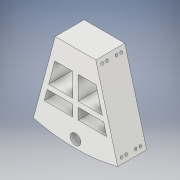
# Autodesk Inventor part: CA001
Saved by Autodesk Inventor 2017 SP1 (Build 210196100, 196)
## iProperties
Created: 2017-06-04
Part Number: CA001
Material: ABS Plastic
Document SubType Name: Modeling
Designer: Zach
Density: 1.06 g/cm^3
Appearance: CR White
Author: Zach
Autodesk Inventor part; units mm, degrees
ref_plane "YZ Plane" through (0, 0, 0) normal (1, 0, 0) x (0, 1, 0)
ref_plane "XZ Plane" through (0, 0, 0) normal (0, 1, 0) x (-1, 0, 0)
ref_plane "XY Plane" through (0, 0, 0) normal (0, 0, 1) x (1, 0, 0)
sketch "Sketch1" plane through (0, 0, 0) normal (0, 0, 1) x (1, 0, 0)
  line L0 (0, 0) -> (160, 0)
  line L1 (160, 0) -> (118.589, 154.5481)
  line L2 (41.411, 154.5481) -> (0, 0)
  line L3 (41.411, 154.5481) -> (118.589, 154.5481)
  dimension "d0" = 160
  dimension "d1" = 160
  dimension "d2" = 75
  dimension "d8" = 75
  constraints: 8 end point, 2 horizontal
  measures "d0" distance of L0.start L0.end
  measures "d1" distance of L1.end L0.end
  measures "d2" angle of L1 L0
  measures "d8" angle of L0 L2
extrude "Extrusion1" add sketch "Sketch1" along normal blind 55
sketch "Sketch6" plane through (0, 0, 55) normal (0, 0, 1) x (1, 0, 0)
  line L0 (0, 0) -> (160, 0) construction
  line L1 (160, 0) -> (118.589, 154.5481) construction
  line L2 (118.589, 154.5481) -> (41.411, 154.5481) construction
  line L3 (41.411, 154.5481) -> (0, 0) construction
  line L4 (110.9157, 144.5481) -> (146.9677, 10) construction
  line L5 (146.9677, 10) -> (13.0323, 10) construction
  line L6 (13.0323, 10) -> (49.0843, 144.5481) construction
  line L7 (49.0843, 144.5481) -> (110.9157, 144.5481) construction
  line L8 (85, 144.5481) -> (75, 144.5481) construction
  line L9 (75, 144.5481) -> (75, 10) construction
  line L10 (75, 10) -> (85, 10) construction
  line L11 (85, 10) -> (85, 144.5481) construction
  line L12 (133.5703, 60) -> (26.4297, 60) construction
  line L13 (26.4297, 60) -> (26.4297, 70) construction
  line L14 (26.4297, 70) -> (133.5703, 70) construction
  line L15 (133.5703, 70) -> (133.5703, 60) construction
  line L16 (133.5703, 60) -> (146.9677, 10)
  line L17 (85, 10) -> (146.9677, 10)
  line L18 (0, 0) -> (160, 0) construction
  line L19 (133.5703, 60) -> (85, 60)
  line L20 (85, 60) -> (85, 10)
  line L21 (75, 10) -> (75, 60)
  line L22 (26.4297, 60) -> (75, 60)
  line L23 (26.4297, 60) -> (13.0323, 10)
  line L24 (13.0323, 10) -> (75, 10)
  line L25 (75, 70) -> (75, 144.5481)
  line L26 (75, 144.5481) -> (49.0843, 144.5481)
  line L27 (75, 70) -> (29.1092, 70)
  line L28 (29.1092, 70) -> (49.0843, 144.5481)
  line L29 (85, 144.5481) -> (110.9157, 144.5481)
  line L30 (110.9157, 144.5481) -> (130.8908, 70)
  line L31 (130.8908, 70) -> (85, 70)
  line L32 (85, 70) -> (85, 144.5481)
  point P0 (80, 10)
  dimension "d22" = 10
  dimension "d23" = 10
  dimension "d24" = 10
  dimension "d25" = 50
  constraints: 56 end point, 16 point on line, 6 collinear, 6 parallel, 3 perpendicular, 2 horizontal, 2 midpoint, 3 other
  measures "d22" distance between parallel lines of L1 L4
  measures "d23" distance between parallel lines of L9 L11
  measures "d24" distance of L12.end L13.end
  measures "d25" distance between parallel lines of L5 L12
extrude "Extrusion5" cut sketch "Sketch6" against normal through all
sketch "Sketch7" plane through (0, 0, 0) normal (0, 0, -1) x (-1, 0, 0)
  circle A0 centre (-80, 304.672) radius 315 construction
  line L0 (0, 0) -> (-160, 0) projected
  arc A1 (-160, 0) -> (0, 0) centre (-80, 304.672) ccw
  dimension "d28" = 630
  constraints: 4 point on circle, 2 centre point, 1 concentric
  measures "d28" diameter of A0
extrude "Extrusion6" add sketch "Sketch7" against normal blind 55
sketch "Sketch8" plane through (0, 0, 0) normal (0, 0, -1) x (-1, 0, 0)
  circle A0 centre (-80, 4.836) radius 10
  line L0 (-15.7117, 20) -> (-144.2883, 20) construction
  line L1 (-13.0323, 10) -> (-15.7117, 20)
  line L2 (-15.7117, 20) -> (-75, 20)
  line L3 (-75, 10) -> (-75, 60) projected
  line L4 (-75, 20) -> (-75, 10)
  line L5 (-75, 10) -> (-13.0323, 10) projected
  line L6 (-75, 10) -> (-13.0323, 10)
  line L7 (-26.4297, 60) -> (-13.0323, 10) projected
  line L8 (-85, 10) -> (-146.9677, 10) projected
  line L9 (-146.9677, 10) -> (-144.2883, 20)
  line L10 (-133.5703, 60) -> (-146.9677, 10) projected
  line L11 (-144.2883, 20) -> (-85, 20)
  line L12 (-85, 60) -> (-85, 10) projected
  line L13 (-85, 20) -> (-85, 10)
  line L14 (-85, 10) -> (-146.9677, 10)
  line L15 (-118.589, 154.5481) -> (-41.411, 154.5481) projected
  arc A1 (-160, 0) -> (0, 0) centre (-80, 304.672) ccw projected
  line L16 (0, -10.328) -> (-160, -10.328) construction
  arc A2 (-160, 0) -> (0, 0) centre (-80, 304.672) ccw projected
  line L17 (-0.263, 4.836) -> (-159.737, 4.836) construction
  point P0 (-80, 154.5481)
  dimension "d31" = 20
  dimension "d32" = 20
  constraints: 22 end point, 6 point on line, 4 collinear, 3 horizontal, 2 midpoint, 1 centre point, 1 coincident, 1 perpendicular, 1 tangent, 1 vertical alignment, 1 other
  measures "d31" diameter of A0
  measures "d32" distance from line of A1.end L0
extrude "Extrusion8" add sketch "Sketch8" against normal blind 55 contours L5 L3 A0 | A0 L3 L2 L1 L5 | L8 L9 L11 L12 A0 | A0 L12 L8
extrude "Extrusion7" cut sketch "Sketch8" against normal through all contours A0 L8 L12 L3 L5 | L5 L3 A0 | A0 L12 L8
sketch "Sketch14" plane through (15.7117, 20, 0) normal (0, 1, 0) x (1, 0, 0)
  line L0 (0, 0) -> (59.2883, 0) construction
  line L1 (0, -55) -> (0, 0) construction
  line L2 (59.2883, -55) -> (0, -55) construction
  line L3 (59.2883, 0) -> (59.2883, -55) construction
  line L4 (69.2883, 0) -> (128.5765, 0) construction
  line L5 (69.2883, -55) -> (69.2883, 0) construction
  line L6 (128.5765, -55) -> (69.2883, -55) construction
  line L7 (128.5765, 0) -> (128.5765, -55) construction
  circle A0 centre (118.9324, -7.5) radius 2.5
  circle A1 centre (78.9324, -7.5) radius 2.5
  circle A2 centre (78.9324, -47.5) radius 2.5
  circle A3 centre (118.9324, -47.5) radius 2.5
  line L8 (118.9324, -7.5) -> (78.9324, -7.5) construction
  line L9 (78.9324, -7.5) -> (78.9324, -47.5) construction
  line L10 (78.9324, -47.5) -> (118.9324, -47.5) construction
  line L11 (118.9324, -47.5) -> (118.9324, -7.5) construction
  line L12 (49.6441, -7.5) -> (9.6441, -7.5) construction
  line L13 (9.6441, -7.5) -> (9.6441, -47.5) construction
  line L14 (9.6441, -47.5) -> (49.6441, -47.5) construction
  line L15 (49.6441, -47.5) -> (49.6441, -7.5) construction
  circle A4 centre (49.6441, -7.5) radius 2.5
  circle A5 centre (9.6441, -7.5) radius 2.5
  circle A6 centre (9.6441, -47.5) radius 2.5
  circle A7 centre (49.6441, -47.5) radius 2.5
  point P0 (-15.7117, 0)
  point P1 (78.9324, -27.5)
  point P2 (98.9324, -7.5)
  point P3 (29.6441, -7.5)
  point P4 (49.6441, -27.5)
  dimension "d77" = 5
  dimension "d78" = 5
  dimension "d79" = 5
  dimension "d80" = 5
  dimension "d81" = 40
  dimension "d83" = 40
  dimension "d84" = 40
  dimension "d85" = 40
  dimension "d86" = 5
  dimension "d87" = 5
  dimension "d88" = 5
  dimension "d89" = 5
  constraints: 16 end point, 8 centre point, 6 coincident, 4 midpoint, 4 parallel, 2 horizontal, 2 perpendicular
  measures "d77" diameter of A0
  measures "d78" diameter of A1
  measures "d79" diameter of A2
  measures "d80" diameter of A3
  measures "d81" distance of L8.start L8.end
  measures "d83" distance of L10.end L8.start
  measures "d84" distance of L14.end L13.end
  measures "d85" distance of L13.end L12.end
  measures "d86" diameter of A4
  measures "d87" diameter of A5
  measures "d88" diameter of A6
  measures "d89" diameter of A7
extrude "Extrusion14" cut sketch "Sketch14" against normal through all
sketch "Sketch15" plane through (0, 0, 55) normal (0, 0, 1) x (1, 0, 0)
  line L0 (75, 20) -> (15.7117, 20) projected
  line L1 (15.7117, 20) -> (144.2883, 20)
  line L2 (144.2883, 20) -> (144.2883, 39)
  line L3 (144.2883, 39) -> (15.7117, 39)
  line L4 (15.7117, 39) -> (15.7117, 20)
  line L5 (40.899, 114) -> (119.101, 114)
  line L6 (119.101, 114) -> (119.101, 144.5481)
  line L7 (119.101, 144.5481) -> (40.899, 144.5481)
  line L8 (40.899, 144.5481) -> (40.899, 114)
  line L9 (110.9157, 144.5481) -> (130.8908, 70) projected
  line L10 (29.1092, 70) -> (49.0843, 144.5481) projected
  point P0 (0, 0)
  dimension "d92" = 19
  dimension "d93" = 30.5481
  constraints: 16 end point, 4 parallel, 2 horizontal, 2 perpendicular, 2 point on line, 1 coincident, 1 horizontal alignment
  measures "d92" distance of L2.end L1.end
  measures "d93" distance of L5.end L6.end
extrude "Extrusion15" add sketch "Sketch15" against normal blind 55
sketch "Sketch10" plane through (41.411, 154.5481, 0) normal (-0.9659, 0.2588, 0) x (0, 0, 1)
  line L0 (9.525, -9.525) -> (9.525, -150.475) construction
  line L1 (0, 0) -> (0, -160) projected
  circle A0 centre (9.525, -150.475) radius 2.5
  circle A1 centre (9.525, -9.525) radius 2.5
  line L2 (45.475, -9.525) -> (45.475, -150.475) construction
  line L3 (55, 0) -> (55, -160) projected
  circle A2 centre (45.475, -150.475) radius 2.5
  circle A3 centre (45.475, -9.525) radius 2.5
  point P0 (9.525, -80)
  point P1 (0, -80)
  dimension "d41" = 140.95
  dimension "d42" = 9.525
  dimension "d43" = 5
  dimension "d44" = 5
  dimension "d45" = 9.525
  dimension "d46" = 5
  dimension "d47" = 5
  constraints: 4 centre point, 4 coincident, 4 end point, 3 horizontal alignment, 2 midpoint, 2 vertical
  measures "d41" distance of L0.start L0.end
  measures "d42" distance between parallel lines of L1 L0
  measures "d43" diameter of A0
  measures "d44" diameter of A1
  measures "d45" distance between parallel lines of L3 L2
  measures "d46" diameter of A2
  measures "d47" diameter of A3
extrude "Extrusion10" cut sketch "Sketch10" against normal blind 25
sketch "Sketch13" plane through (41.411, 154.5481, 0) normal (-0.9659, 0.2588, 0) x (0, 0, 1)
  line L0 (18.4199, -9.525) -> (18.4199, -150.475) construction
  line L1 (36.5801, -9.525) -> (36.5801, -150.475) construction
  line L2 (0, 0) -> (0, -160) construction
  line L3 (55, 0) -> (55, -160) construction
  circle A0 centre (36.5801, -9.525) radius 2.5
  circle A1 centre (18.4199, -9.525) radius 2.5
  circle A2 centre (36.5801, -150.475) radius 2.5
  circle A3 centre (18.4199, -150.475) radius 2.5
  point P0 (18.4199, -80)
  point P1 (0, -80)
  point P2 (55, -80)
  point P3 (36.5801, -80)
  dimension "d68" = 140.95
  dimension "d69" = 18.4199
  dimension "d70" = 18.4199
  dimension "d71" = 5
  dimension "d72" = 5
  dimension "d73" = 5
  dimension "d74" = 5
  constraints: 4 centre point, 4 coincident, 4 end point, 4 horizontal alignment, 4 midpoint, 2 vertical
  measures "d68" distance of L0.start L0.end
  measures "d69" distance between parallel lines of L3 L1
  measures "d70" distance between parallel lines of L2 L0
  measures "d71" diameter of A0
  measures "d72" diameter of A1
  measures "d73" diameter of A2
  measures "d74" diameter of A3
extrude "Extrusion13" cut sketch "Sketch13" against normal blind 25
sketch "Sketch11" plane through (118.589, 154.5481, 55) normal (0.9659, 0.2588, 0) x (0, 0, -1)
  line L0 (45.475, -150.475) -> (45.475, -9.525) construction
  line L1 (9.525, -150.475) -> (9.525, -9.525) construction
  line L2 (0, -160) -> (0, 0) projected
  line L3 (55, -160) -> (55, 0) projected
  circle A0 centre (9.525, -9.525) radius 2.5
  circle A1 centre (45.475, -9.525) radius 2.5
  circle A2 centre (45.475, -150.475) radius 2.5
  circle A3 centre (9.525, -150.475) radius 2.5
  point P0 (55, -118.589)
  point P1 (9.525, -80)
  point P2 (0, -80)
  dimension "d50" = 9.525
  dimension "d51" = 9.525
  dimension "d52" = 5
  dimension "d53" = 5
  dimension "d54" = 5
  dimension "d55" = 5
  dimension "d56" = 140.95
  constraints: 4 centre point, 4 coincident, 4 end point, 3 horizontal alignment, 2 midpoint, 2 vertical
  measures "d50" distance between parallel lines of L2 L1
  measures "d51" distance between parallel lines of L3 L0
  measures "d52" diameter of A0
  measures "d53" diameter of A1
  measures "d54" diameter of A2
  measures "d55" diameter of A3
  measures "d56" distance of L1.start L1.end
extrude "Extrusion11" cut sketch "Sketch11" against normal blind 25
sketch "Sketch12" plane through (118.589, 154.5481, 55) normal (0.9659, 0.2588, 0) x (0, 0, -1)
  line L0 (36.5801, -150.475) -> (36.5801, -9.525) construction
  line L1 (55, -160) -> (55, 0) construction
  line L2 (18.4199, -150.475) -> (18.4199, -9.525) construction
  line L3 (0, -160) -> (0, 0) construction
  circle A0 centre (18.4199, -150.475) radius 2.5
  circle A1 centre (36.5801, -150.475) radius 2.5
  circle A2 centre (36.5801, -9.525) radius 2.5
  circle A3 centre (18.4199, -9.525) radius 2.5
  point P0 (55, -118.589)
  point P1 (18.4199, -80)
  point P2 (0, -80)
  dimension "d59" = 18.4199
  dimension "d60" = 18.4199
  dimension "d61" = 5
  dimension "d62" = 5
  dimension "d63" = 5
  dimension "d64" = 5
  dimension "d65" = 140.95
  constraints: 4 centre point, 4 coincident, 4 end point, 3 horizontal alignment, 2 midpoint, 2 vertical
  measures "d59" distance between parallel lines of L1 L0
  measures "d60" distance between parallel lines of L3 L2
  measures "d61" diameter of A0
  measures "d62" diameter of A1
  measures "d63" diameter of A2
  measures "d64" diameter of A3
  measures "d65" distance of L0.start L0.end
extrude "Extrusion12" cut sketch "Sketch12" against normal blind 25
equation "\"d83\" = d81"
equation "\"d84\" = d81"
equation "\"d85\" = d81"
body "Solid1"
